Autodesk Inventor part; units mm, degrees
(part 2 of 2)
  arc A595 (0.658, -32.4933) -> (0.5633, -32.568) centre (0.66, -32.5933) ccw
  arc A596 (-0.2221, -33.5687) -> (-0.1304, -33.6297) centre (-0.13, -33.5297) ccw
  arc A597 (-0.5633, -32.568) -> (-0.2221, -33.5687) centre (6.5366, -30.706) ccw
  arc A598 (-0.5633, -32.568) -> (-0.658, -32.4933) centre (-0.66, -32.5933) ccw
  arc A599 (0.2221, -33.5687) -> (0.5633, -32.568) centre (-6.5366, -30.706) ccw
  arc A600 (0.1304, -33.6297) -> (0.2221, -33.5687) centre (0.13, -33.5297) ccw
  arc A601 (2.2033, -32.4252) -> (2.1123, -32.5043) centre (2.2101, -32.525) ccw
  arc A602 (1.3754, -33.5413) -> (1.4699, -33.5979) centre (1.4656, -33.498) ccw
  arc A603 (0.987, -32.5579) -> (1.3754, -33.5413) centre (7.9903, -30.3602) ccw
  arc A604 (0.987, -32.5579) -> (0.8889, -32.4878) centre (0.8916, -32.5878) ccw
  arc A605 (1.8191, -33.5202) -> (2.1123, -32.5043) centre (-5.0682, -30.9823) ccw
  arc A606 (1.7304, -33.5855) -> (1.8191, -33.5202) centre (1.7253, -33.4856) ccw
  arc A607 (3.7437, -32.2837) -> (3.6565, -32.3669) centre (3.7552, -32.383) ccw
  arc A608 (2.9698, -33.4379) -> (3.0669, -33.4899) centre (3.0578, -33.3903) ccw
  arc A609 (2.5351, -32.474) -> (2.9698, -33.4379) centre (9.4258, -29.9456) ccw
  arc A610 (2.5351, -32.474) -> (2.4337, -32.4088) centre (2.4412, -32.5085) ccw
  arc A611 (3.412, -33.3956) -> (3.6565, -32.3669) centre (-3.5883, -31.1883) ccw
  arc A612 (3.3265, -33.4651) -> (3.412, -33.3956) centre (3.3166, -33.3656) ccw
  arc A613 (5.2756, -32.069) -> (5.1924, -32.1563) centre (5.2918, -32.1676) ccw
  arc A614 (4.5575, -33.2587) -> (4.657, -33.306) centre (4.6431, -33.207) ccw
  arc A615 (4.0774, -32.3166) -> (4.5575, -33.2587) centre (10.84, -29.4632) ccw
  arc A616 (4.0774, -32.3166) -> (3.973, -32.2562) centre (3.9852, -32.3555) ccw
  arc A617 (4.9972, -33.1955) -> (5.1924, -32.1563) centre (-2.1002, -31.3237) ccw
  arc A618 (4.9151, -33.2689) -> (4.9972, -33.1955) centre (4.9005, -33.17) ccw
  arc A619 (6.7955, -31.7816) -> (6.7166, -31.8728) centre (6.8164, -31.8794) ccw
  arc A620 (6.1349, -33.0041) -> (6.2364, -33.0467) centre (6.2179, -32.9484) ccw
  arc A621 (5.6104, -32.086) -> (6.1349, -33.0041) centre (12.2297, -28.9141) ccw
  arc A622 (5.6104, -32.086) -> (5.5033, -32.0307) centre (5.5203, -32.1292) ccw
  arc A623 (6.571, -32.9201) -> (6.7166, -31.8728) centre (-0.6074, -31.3882) ccw
  arc A624 (6.4925, -32.9973) -> (6.571, -32.9201) centre (6.4732, -32.8992) ccw
  arc A625 (8.3, -31.4223) -> (8.2256, -31.5171) centre (8.3256, -31.519) ccw
  arc A626 (7.6983, -32.6749) -> (7.8018, -32.7125) centre (7.7786, -32.6152) ccw
  arc A627 (7.1308, -31.7827) -> (7.6983, -32.6749) centre (13.5916, -28.2994) ccw
  arc A628 (7.1308, -31.7827) -> (7.0212, -31.7325) centre (7.0428, -31.8302) ccw
  arc A629 (8.13, -32.5701) -> (8.2256, -31.5171) centre (0.8868, -31.3815) ccw
  arc A630 (8.0552, -32.651) -> (8.13, -32.5701) centre (8.0313, -32.5539) ccw
  arc A631 (9.7858, -30.9918) -> (9.7159, -31.09) centre (9.8159, -31.0871) ccw
  arc A632 (9.2443, -32.2715) -> (9.3495, -32.3042) centre (9.3217, -32.2082) ccw
  arc A633 (8.635, -31.4074) -> (9.2443, -32.2715) centre (14.9228, -27.6206) ccw
  arc A634 (8.635, -31.4074) -> (8.5231, -31.3625) centre (8.5493, -31.459) ccw
  arc A635 (9.6705, -32.1464) -> (9.7159, -31.09) centre (2.379, -31.3038) ccw
  arc A636 (9.5997, -32.2308) -> (9.6705, -32.1464) centre (9.5712, -32.1349) ccw
  arc A637 (11.2493, -30.491) -> (11.1842, -30.5925) centre (11.2839, -30.5848) ccw
  arc A638 (10.7694, -31.7951) -> (10.876, -31.8228) centre (10.8437, -31.7282) ccw
  arc A639 (10.1196, -30.961) -> (10.7694, -31.7951) centre (16.2201, -26.8793) ccw
  arc A640 (10.1196, -30.961) -> (10.0057, -30.9214) centre (10.0365, -31.0166) ccw
  arc A641 (11.1891, -31.6499) -> (11.1842, -30.5925) centre (3.8658, -31.1551) ccw
  arc A642 (11.1224, -31.7375) -> (11.1891, -31.6499) centre (11.0894, -31.6431) ccw
  arc A643 (12.6874, -29.9212) -> (12.6272, -30.0257) centre (12.7264, -30.0133) ccw
  arc A644 (12.2701, -31.2467) -> (12.3779, -31.2692) centre (12.3411, -31.1763) ccw
  arc A645 (11.5814, -30.4444) -> (12.2701, -31.2467) centre (17.4807, -26.0771) ccw
  arc A646 (11.5814, -30.4444) -> (11.4657, -30.4103) centre (11.501, -30.5039) ccw
  arc A647 (12.6824, -31.0816) -> (12.6272, -30.0257) centre (5.3439, -30.9359) ccw
  arc A648 (12.62, -31.1723) -> (12.6824, -31.0816) centre (12.5824, -31.0796) ccw
  arc A649 (14.0967, -29.2836) -> (14.0416, -29.3909) centre (14.1401, -29.3738) ccw
  arc A650 (13.743, -30.6275) -> (13.8517, -30.6449) centre (13.8105, -30.5537) ccw
  arc A651 (13.0168, -29.8588) -> (13.743, -30.6275) centre (18.7017, -25.2158) ccw
  arc A652 (13.0168, -29.8588) -> (12.8997, -29.8303) centre (12.9394, -29.9221) ccw
  arc A653 (14.147, -30.443) -> (14.0416, -29.3909) centre (6.8098, -30.6466) ccw
  arc A654 (14.0889, -30.5365) -> (14.147, -30.443) centre (14.047, -30.4457) ccw
  arc A655 (15.4741, -28.5797) -> (15.4242, -28.6894) centre (15.5218, -28.6677) ccw
  arc A656 (15.1847, -29.9389) -> (15.2941, -29.9511) centre (15.2487, -29.862) ccw
  arc A657 (14.4228, -29.2057) -> (15.1847, -29.9389) centre (19.8803, -24.2973) ccw
  arc A658 (14.4228, -29.2057) -> (14.3045, -29.1827) centre (14.3485, -29.2725) ccw
  arc A659 (15.5795, -29.7353) -> (15.4242, -28.6894) centre (8.2603, -30.2879) ccw
  arc A660 (15.5259, -29.8316) -> (15.5795, -29.7353) centre (15.4798, -29.7429) ccw
  arc A661 (16.8165, -27.8111) -> (16.7718, -27.923) centre (16.8682, -27.8966) ccw
  arc A662 (16.592, -29.1824) -> (16.702, -29.1894) centre (16.6523, -29.1026) ccw
  arc A663 (15.7962, -28.4863) -> (16.592, -29.1824) centre (21.0139, -23.3239) ccw
  arc A664 (15.7962, -28.4863) -> (15.6768, -28.469) centre (15.7251, -28.5566) ccw
  arc A665 (16.9767, -28.9603) -> (16.7718, -27.923) centre (9.6921, -29.8605) ccw
  arc A666 (16.9278, -29.059) -> (16.9767, -28.9603) centre (16.8775, -28.9726) ccw
  arc A667 (18.1207, -26.9794) -> (18.0814, -27.0934) centre (18.1765, -27.0624) ccw
  arc A668 (17.9618, -28.3599) -> (18.0719, -28.3616) centre (18.0182, -28.2773) ccw
  arc A669 (17.1337, -27.7024) -> (17.9618, -28.3599) centre (22.0999, -22.2976) ccw
  arc A670 (17.1337, -27.7024) -> (17.0137, -27.6909) centre (17.0661, -27.7761) ccw
  arc A671 (18.3355, -28.1198) -> (18.0814, -27.0934) centre (11.102, -29.3655) ccw
  arc A672 (18.2913, -28.2207) -> (18.3355, -28.1198) centre (18.2369, -28.1367) ccw
  arc A673 (19.384, -26.0866) -> (19.3501, -26.2023) centre (19.4436, -26.1669) ccw
  arc A674 (19.2909, -27.4731) -> (19.401, -27.4696) centre (19.3433, -27.3879) ccw
  arc A675 (18.4324, -26.8558) -> (19.2909, -27.4731) centre (23.1358, -21.2208) ccw
  arc A676 (18.4324, -26.8558) -> (18.312, -26.85) centre (18.3684, -26.9326) ccw
  arc A677 (19.6527, -27.2155) -> (19.3501, -26.2023) centre (12.4866, -28.804) ccw
  arc A678 (19.6134, -27.3184) -> (19.6527, -27.2155) centre (19.5551, -27.2371) ccw
  arc A679 (20.6033, -25.1348) -> (20.5749, -25.2519) centre (20.6666, -25.2121) ccw
  arc A680 (20.5763, -26.5241) -> (20.686, -26.5154) centre (20.6245, -26.4365) ccw
  arc A681 (19.6894, -25.9483) -> (20.5763, -26.5241) centre (24.1194, -20.0959) ccw
  arc A682 (19.6894, -25.9483) -> (19.5688, -25.9482) centre (19.6291, -26.0281) ccw
  arc A683 (20.9254, -26.2495) -> (20.5749, -25.2519) centre (13.8431, -28.1772) ccw
  arc A684 (20.891, -26.3542) -> (20.9254, -26.2495) centre (20.8289, -26.2758) ccw
  arc A685 (21.7759, -24.1259) -> (21.7532, -24.2444) centre (21.8429, -24.2002) ccw
  arc A686 (21.815, -25.515) -> (21.9243, -25.5011) centre (21.8591, -25.4252) ccw
  arc A687 (20.9018, -24.9821) -> (21.815, -25.515) centre (25.0482, -18.9255) ccw
  arc A688 (20.9018, -24.9821) -> (20.7813, -24.9877) centre (20.8453, -25.0646) ccw
  arc A689 (22.1507, -25.2241) -> (21.7532, -24.2444) centre (15.1681, -27.4867) ccw
  arc A690 (22.1213, -25.3303) -> (22.1507, -25.2241) centre (22.0556, -25.255) ccw
  arc A691 (22.8992, -23.0625) -> (22.8821, -23.1818) centre (22.9696, -23.1334) ccw
  arc A692 (23.0044, -24.4481) -> (23.1128, -24.429) centre (23.0441, -24.3563) ccw
  arc A693 (22.0668, -23.9592) -> (23.0044, -24.4481) centre (25.9204, -17.7122) ccw
  arc A694 (22.0668, -23.9592) -> (21.9468, -23.9706) centre (22.0143, -24.0443) ccw
  arc A695 (23.3258, -24.1416) -> (22.8821, -23.1818) centre (16.4588, -26.7338) ccw
  arc A696 (23.3015, -24.249) -> (23.3258, -24.1416) centre (23.2323, -24.1769) ccw
  arc A697 (23.9706, -21.9468) -> (23.9592, -22.0668) centre (24.0443, -22.0143) ccw
  arc A698 (24.1416, -23.3258) -> (24.249, -23.3015) centre (24.1769, -23.2323) ccw
  arc A699 (23.1818, -22.8821) -> (24.1416, -23.3258) centre (26.7338, -16.4588) ccw
  arc A700 (23.1818, -22.8821) -> (23.0625, -22.8992) centre (23.1334, -22.9696) ccw
  arc A701 (24.4481, -23.0044) -> (23.9592, -22.0668) centre (17.7122, -25.9204) ccw
  arc A702 (24.429, -23.1128) -> (24.4481, -23.0044) centre (24.3563, -23.0441) ccw
  arc A703 (24.9877, -20.7813) -> (24.9821, -20.9018) centre (25.0646, -20.8453) ccw
  arc A704 (25.2241, -22.1507) -> (25.3303, -22.1213) centre (25.255, -22.0556) ccw
  arc A705 (24.2444, -21.7532) -> (25.2241, -22.1507) centre (27.4867, -15.1681) ccw
  arc A706 (24.2444, -21.7532) -> (24.1259, -21.7759) centre (24.2002, -21.8429) ccw
  arc A707 (25.515, -21.815) -> (24.9821, -20.9018) centre (18.9255, -25.0482) ccw
  arc A708 (25.5011, -21.9243) -> (25.515, -21.815) centre (25.4252, -21.8591) ccw
  arc A709 (25.9482, -19.5688) -> (25.9483, -19.6894) centre (26.0281, -19.6291) ccw
  arc A710 (26.2495, -20.9254) -> (26.3542, -20.891) centre (26.2758, -20.8289) ccw
  arc A711 (25.2519, -20.5749) -> (26.2495, -20.9254) centre (28.1772, -13.8431) ccw
  arc A712 (25.2519, -20.5749) -> (25.1348, -20.6033) centre (25.2121, -20.6666) ccw
  arc A713 (26.5241, -20.5763) -> (25.9483, -19.6894) centre (20.0959, -24.1194) ccw
  arc A714 (26.5154, -20.686) -> (26.5241, -20.5763) centre (26.4365, -20.6245) ccw
  arc A715 (26.85, -18.312) -> (26.8558, -18.4324) centre (26.9326, -18.3684) ccw
  arc A716 (27.2155, -19.6527) -> (27.3184, -19.6134) centre (27.2371, -19.5551) ccw
  arc A717 (26.2023, -19.3501) -> (27.2155, -19.6527) centre (28.804, -12.4866) ccw
  arc A718 (26.2023, -19.3501) -> (26.0866, -19.384) centre (26.1669, -19.4436) ccw
  arc A719 (27.4731, -19.2909) -> (26.8558, -18.4324) centre (21.2208, -23.1358) ccw
  arc A720 (27.4696, -19.401) -> (27.4731, -19.2909) centre (27.3879, -19.3433) ccw
  arc A721 (27.6909, -17.0137) -> (27.7024, -17.1337) centre (27.7761, -17.0661) ccw
  arc A722 (28.1198, -18.3355) -> (28.2207, -18.2913) centre (28.1367, -18.2369) ccw
  arc A723 (27.0934, -18.0814) -> (28.1198, -18.3355) centre (29.3655, -11.102) ccw
  arc A724 (27.0934, -18.0814) -> (26.9794, -18.1207) centre (27.0624, -18.1765) ccw
  arc A725 (28.3599, -17.9618) -> (27.7024, -17.1337) centre (22.2976, -22.0999) ccw
  arc A726 (28.3616, -18.0719) -> (28.3599, -17.9618) centre (28.2773, -18.0182) ccw
  arc A727 (28.469, -15.6768) -> (28.4863, -15.7962) centre (28.5566, -15.7251) ccw
  arc A728 (28.9603, -16.9767) -> (29.059, -16.9278) centre (28.9726, -16.8775) ccw
  arc A729 (27.923, -16.7718) -> (28.9603, -16.9767) centre (29.8605, -9.6921) ccw
  arc A730 (27.923, -16.7718) -> (27.8111, -16.8165) centre (27.8966, -16.8682) ccw
  arc A731 (29.1824, -16.592) -> (28.4863, -15.7962) centre (23.3239, -21.0139) ccw
  arc A732 (29.1894, -16.702) -> (29.1824, -16.592) centre (29.1026, -16.6523) ccw
  arc A733 (29.1827, -14.3045) -> (29.2057, -14.4228) centre (29.2725, -14.3485) ccw
  arc A734 (29.7353, -15.5795) -> (29.8316, -15.5259) centre (29.7429, -15.4798) ccw
  arc A735 (28.6894, -15.4242) -> (29.7353, -15.5795) centre (30.2879, -8.2603) ccw
  arc A736 (28.6894, -15.4242) -> (28.5797, -15.4741) centre (28.6677, -15.5218) ccw
  arc A737 (29.9389, -15.1847) -> (29.2057, -14.4228) centre (24.2973, -19.8803) ccw
  arc A738 (29.9511, -15.2941) -> (29.9389, -15.1847) centre (29.862, -15.2487) ccw
  arc A739 (29.8303, -12.8997) -> (29.8588, -13.0168) centre (29.9221, -12.9394) ccw
  arc A740 (30.443, -14.147) -> (30.5365, -14.0889) centre (30.4457, -14.047) ccw
  arc A741 (29.3909, -14.0416) -> (30.443, -14.147) centre (30.6466, -6.8098) ccw
  arc A742 (29.3909, -14.0416) -> (29.2836, -14.0967) centre (29.3738, -14.1401) ccw
  arc A743 (30.6275, -13.743) -> (29.8588, -13.0168) centre (25.2158, -18.7017) ccw
  arc A744 (30.6449, -13.8517) -> (30.6275, -13.743) centre (30.5537, -13.8105) ccw
  arc A745 (30.4103, -11.4657) -> (30.4444, -11.5814) centre (30.5039, -11.501) ccw
  arc A746 (31.0816, -12.6824) -> (31.1723, -12.62) centre (31.0796, -12.5824) ccw
  arc A747 (30.0257, -12.6272) -> (31.0816, -12.6824) centre (30.9359, -5.3439) ccw
  arc A748 (30.0257, -12.6272) -> (29.9212, -12.6874) centre (30.0133, -12.7264) ccw
  arc A749 (31.2467, -12.2701) -> (30.4444, -11.5814) centre (26.0771, -17.4807) ccw
  arc A750 (31.2692, -12.3779) -> (31.2467, -12.2701) centre (31.1763, -12.3411) ccw
  arc A751 (30.9214, -10.0057) -> (30.961, -10.1196) centre (31.0166, -10.0365) ccw
  arc A752 (31.6499, -11.1891) -> (31.7375, -11.1224) centre (31.6431, -11.0894) ccw
  arc A753 (30.5925, -11.1842) -> (31.6499, -11.1891) centre (31.1551, -3.8658) ccw
  arc A754 (30.5925, -11.1842) -> (30.491, -11.2493) centre (30.5848, -11.2839) ccw
  arc A755 (31.7951, -10.7694) -> (30.961, -10.1196) centre (26.8793, -16.2201) ccw
  arc A756 (31.8228, -10.876) -> (31.7951, -10.7694) centre (31.7282, -10.8437) ccw
  arc A757 (31.3625, -8.5231) -> (31.4074, -8.635) centre (31.459, -8.5493) ccw
  arc A758 (32.1464, -9.6705) -> (32.2308, -9.5997) centre (32.1349, -9.5712) ccw
  arc A759 (31.09, -9.7159) -> (32.1464, -9.6705) centre (31.3038, -2.379) ccw
  arc A760 (31.09, -9.7159) -> (30.9918, -9.7858) centre (31.0871, -9.8159) ccw
  arc A761 (32.2715, -9.2443) -> (31.4074, -8.635) centre (27.6206, -14.9228) ccw
  arc A762 (32.3042, -9.3495) -> (32.2715, -9.2443) centre (32.2082, -9.3217) ccw
  arc A763 (31.7325, -7.0212) -> (31.7827, -7.1308) centre (31.8302, -7.0428) ccw
  arc A764 (32.5701, -8.13) -> (32.651, -8.0552) centre (32.5539, -8.0313) ccw
  arc A765 (31.5171, -8.2256) -> (32.5701, -8.13) centre (31.3815, -0.8868) ccw
  arc A766 (31.5171, -8.2256) -> (31.4223, -8.3) centre (31.519, -8.3256) ccw
  arc A767 (32.6749, -7.6983) -> (31.7827, -7.1308) centre (28.2994, -13.5916) ccw
  arc A768 (32.7125, -7.8018) -> (32.6749, -7.6983) centre (32.6152, -7.7786) ccw
  arc A769 (32.0307, -5.5033) -> (32.086, -5.6104) centre (32.1292, -5.5203) ccw
  arc A770 (32.9201, -6.571) -> (32.9973, -6.4925) centre (32.8992, -6.4732) ccw
  arc A771 (31.8728, -6.7166) -> (32.9201, -6.571) centre (31.3882, 0.6074) ccw
  arc A772 (31.8728, -6.7166) -> (31.7816, -6.7955) centre (31.8794, -6.8164) ccw
  arc A773 (33.0041, -6.1349) -> (32.086, -5.6104) centre (28.9141, -12.2297) ccw
  arc A774 (33.0467, -6.2364) -> (33.0041, -6.1349) centre (32.9484, -6.2179) ccw
  arc A775 (32.2562, -3.973) -> (32.3166, -4.0774) centre (32.3555, -3.9852) ccw
  arc A776 (33.1955, -4.9972) -> (33.2689, -4.9151) centre (33.17, -4.9005) ccw
  arc A777 (32.1563, -5.1924) -> (33.1955, -4.9972) centre (31.3237, 2.1002) ccw
  arc A778 (32.1563, -5.1924) -> (32.069, -5.2756) centre (32.1676, -5.2918) ccw
  arc A779 (33.2587, -4.5575) -> (32.3166, -4.0774) centre (29.4632, -10.84) ccw
  arc A780 (33.306, -4.657) -> (33.2587, -4.5575) centre (33.207, -4.6431) ccw
  arc A781 (32.4088, -2.4337) -> (32.474, -2.5351) centre (32.5085, -2.4412) ccw
  arc A782 (33.3956, -3.412) -> (33.4651, -3.3265) centre (33.3656, -3.3166) ccw
  arc A783 (32.3669, -3.6565) -> (33.3956, -3.412) centre (31.1883, 3.5883) ccw
  arc A784 (32.3669, -3.6565) -> (32.2837, -3.7437) centre (32.383, -3.7552) ccw
  arc A785 (33.4379, -2.9698) -> (32.474, -2.5351) centre (29.9456, -9.4258) ccw
  arc A786 (33.4899, -3.0669) -> (33.4379, -2.9698) centre (33.3903, -3.0578) ccw
  arc A787 (32.4878, -0.8889) -> (32.5579, -0.987) centre (32.5878, -0.8916) ccw
  arc A788 (33.5202, -1.8191) -> (33.5855, -1.7304) centre (33.4856, -1.7253) ccw
  arc A789 (32.5043, -2.1123) -> (33.5202, -1.8191) centre (30.9823, 5.0682) ccw
  arc A790 (32.5043, -2.1123) -> (32.4252, -2.2033) centre (32.525, -2.2101) ccw
  arc A791 (33.5413, -1.3754) -> (32.5579, -0.987) centre (30.3602, -7.9903) ccw
  arc A792 (33.5979, -1.4699) -> (33.5413, -1.3754) centre (33.498, -1.4656) ccw
  arc A793 (30.6449, 13.8517) -> (30.5365, 14.0889) centre (0, 0) ccw
  arc A794 (31.2692, 12.3779) -> (31.1723, 12.62) centre (0, 0) ccw
  arc A795 (31.8228, 10.876) -> (31.7375, 11.1224) centre (0, 0) ccw
  arc A796 (32.3042, 9.3495) -> (32.2308, 9.5997) centre (0, 0) ccw
  arc A797 (29.9212, 12.6874) -> (29.8303, 12.8997) centre (0, 0) ccw
  arc A798 (30.491, 11.2493) -> (30.4103, 11.4657) centre (0, 0) ccw
  arc A799 (30.9918, 9.7858) -> (30.9214, 10.0057) centre (0, 0) ccw
  arc A800 (31.4223, 8.3) -> (31.3625, 8.5231) centre (0, 0) ccw
  arc A801 (32.7125, 7.8018) -> (32.651, 8.0552) centre (0, 0) ccw
  arc A802 (33.0467, 6.2364) -> (32.9973, 6.4925) centre (0, 0) ccw
  arc A803 (33.306, 4.657) -> (33.2689, 4.9151) centre (0, 0) ccw
  arc A804 (33.4899, 3.0669) -> (33.4651, 3.3265) centre (0, 0) ccw
  arc A805 (33.5979, 1.4699) -> (33.5855, 1.7304) centre (0, 0) ccw
  arc A806 (33.6297, -0.1304) -> (33.6297, 0.1304) centre (0, 0) ccw
  arc A807 (33.5855, -1.7304) -> (33.5979, -1.4699) centre (0, 0) ccw
  arc A808 (33.4651, -3.3265) -> (33.4899, -3.0669) centre (0, 0) ccw
  arc A809 (31.7816, 6.7955) -> (31.7325, 7.0212) centre (0, 0) ccw
  arc A810 (32.069, 5.2756) -> (32.0307, 5.5033) centre (0, 0) ccw
  arc A811 (32.2837, 3.7437) -> (32.2562, 3.973) centre (0, 0) ccw
  arc A812 (32.4252, 2.2033) -> (32.4088, 2.4337) centre (0, 0) ccw
  arc A813 (32.4933, 0.658) -> (32.4878, 0.8889) centre (0, 0) ccw
  arc A814 (32.4878, -0.8889) -> (32.4933, -0.658) centre (0, 0) ccw
  arc A815 (32.4088, -2.4337) -> (32.4252, -2.2033) centre (0, 0) ccw
  arc A816 (32.2562, -3.973) -> (32.2837, -3.7437) centre (0, 0) ccw
  arc A817 (32.0307, -5.5033) -> (32.069, -5.2756) centre (0, 0) ccw
  arc A818 (31.7325, -7.0212) -> (31.7816, -6.7955) centre (0, 0) ccw
  arc A819 (31.3625, -8.5231) -> (31.4223, -8.3) centre (0, 0) ccw
  arc A820 (30.9214, -10.0057) -> (30.9918, -9.7858) centre (0, 0) ccw
  arc A821 (30.4103, -11.4657) -> (30.491, -11.2493) centre (0, 0) ccw
  arc A822 (29.8303, -12.8997) -> (29.9212, -12.6874) centre (0, 0) ccw
  arc A823 (29.1827, -14.3045) -> (29.2836, -14.0967) centre (0, 0) ccw
  arc A824 (28.469, -15.6768) -> (28.5797, -15.4741) centre (0, 0) ccw
  arc A825 (27.6909, -17.0137) -> (27.8111, -16.8165) centre (0, 0) ccw
  arc A826 (26.85, -18.312) -> (26.9794, -18.1207) centre (0, 0) ccw
  arc A827 (25.9482, -19.5688) -> (26.0866, -19.384) centre (0, 0) ccw
  arc A828 (24.9877, -20.7813) -> (25.1348, -20.6033) centre (0, 0) ccw
  arc A829 (23.9706, -21.9468) -> (24.1259, -21.7759) centre (0, 0) ccw
  arc A830 (22.8992, -23.0625) -> (23.0625, -22.8992) centre (0, 0) ccw
  arc A831 (33.2689, -4.9151) -> (33.306, -4.657) centre (0, 0) ccw
  arc A832 (32.9973, -6.4925) -> (33.0467, -6.2364) centre (0, 0) ccw
  arc A833 (32.651, -8.0552) -> (32.7125, -7.8018) centre (0, 0) ccw
  arc A834 (32.2308, -9.5997) -> (32.3042, -9.3495) centre (0, 0) ccw
  arc A835 (31.7375, -11.1224) -> (31.8228, -10.876) centre (0, 0) ccw
  arc A836 (31.1723, -12.62) -> (31.2692, -12.3779) centre (0, 0) ccw
  arc A837 (30.5365, -14.0889) -> (30.6449, -13.8517) centre (0, 0) ccw
  arc A838 (29.8316, -15.5259) -> (29.9511, -15.2941) centre (0, 0) ccw
  arc A839 (29.059, -16.9278) -> (29.1894, -16.702) centre (0, 0) ccw
  arc A840 (28.2207, -18.2913) -> (28.3616, -18.0719) centre (0, 0) ccw
  arc A841 (27.3184, -19.6134) -> (27.4696, -19.401) centre (0, 0) ccw
  arc A842 (26.3542, -20.891) -> (26.5154, -20.686) centre (0, 0) ccw
  arc A843 (25.3303, -22.1213) -> (25.5011, -21.9243) centre (0, 0) ccw
  arc A844 (24.249, -23.3015) -> (24.429, -23.1128) centre (0, 0) ccw
  arc A845 (23.1128, -24.429) -> (23.3015, -24.249) centre (0, 0) ccw
  arc A846 (21.9243, -25.5011) -> (22.1213, -25.3303) centre (0, 0) ccw
  arc A847 (20.686, -26.5154) -> (20.891, -26.3542) centre (0, 0) ccw
  arc A848 (19.401, -27.4696) -> (19.6134, -27.3184) centre (0, 0) ccw
  arc A849 (18.0719, -28.3616) -> (18.2913, -28.2207) centre (0, 0) ccw
  arc A850 (16.702, -29.1894) -> (16.9278, -29.059) centre (0, 0) ccw
  arc A851 (15.2941, -29.9511) -> (15.5259, -29.8316) centre (0, 0) ccw
  arc A852 (13.8517, -30.6449) -> (14.0889, -30.5365) centre (0, 0) ccw
  arc A853 (12.3779, -31.2692) -> (12.62, -31.1723) centre (0, 0) ccw
  arc A854 (10.876, -31.8228) -> (11.1224, -31.7375) centre (0, 0) ccw
  arc A855 (9.3495, -32.3042) -> (9.5997, -32.2308) centre (0, 0) ccw
  arc A856 (7.8018, -32.7125) -> (8.0552, -32.651) centre (0, 0) ccw
  arc A857 (6.2364, -33.0467) -> (6.4925, -32.9973) centre (0, 0) ccw
  arc A858 (4.657, -33.306) -> (4.9151, -33.2689) centre (0, 0) ccw
  arc A859 (3.0669, -33.4899) -> (3.3265, -33.4651) centre (0, 0) ccw
  arc A860 (1.4699, -33.5979) -> (1.7304, -33.5855) centre (0, 0) ccw
  arc A861 (21.7759, -24.1259) -> (21.9468, -23.9706) centre (0, 0) ccw
  arc A862 (20.6033, -25.1348) -> (20.7813, -24.9877) centre (0, 0) ccw
  arc A863 (19.384, -26.0866) -> (19.5688, -25.9482) centre (0, 0) ccw
  arc A864 (18.1207, -26.9794) -> (18.312, -26.85) centre (0, 0) ccw
  arc A865 (16.8165, -27.8111) -> (17.0137, -27.6909) centre (0, 0) ccw
  arc A866 (15.4741, -28.5797) -> (15.6768, -28.469) centre (0, 0) ccw
  arc A867 (14.0967, -29.2836) -> (14.3045, -29.1827) centre (0, 0) ccw
  arc A868 (12.6874, -29.9212) -> (12.8997, -29.8303) centre (0, 0) ccw
  arc A869 (11.2493, -30.491) -> (11.4657, -30.4103) centre (0, 0) ccw
  arc A870 (9.7858, -30.9918) -> (10.0057, -30.9214) centre (0, 0) ccw
  arc A871 (8.3, -31.4223) -> (8.5231, -31.3625) centre (0, 0) ccw
  arc A872 (6.7955, -31.7816) -> (7.0212, -31.7325) centre (0, 0) ccw
  arc A873 (5.2756, -32.069) -> (5.5033, -32.0307) centre (0, 0) ccw
  arc A874 (3.7437, -32.2837) -> (3.973, -32.2562) centre (0, 0) ccw
  arc A875 (2.2033, -32.4252) -> (2.4337, -32.4088) centre (0, 0) ccw
  arc A876 (0.658, -32.4933) -> (0.8889, -32.4878) centre (0, 0) ccw
  arc A877 (-0.8889, -32.4878) -> (-0.658, -32.4933) centre (0, 0) ccw
  arc A878 (-0.1304, -33.6297) -> (0.1304, -33.6297) centre (0, 0) ccw
  arc A879 (-1.7304, -33.5855) -> (-1.4699, -33.5979) centre (0, 0) ccw
  arc A880 (-3.3265, -33.4651) -> (-3.0669, -33.4899) centre (0, 0) ccw
  arc A881 (-4.9151, -33.2689) -> (-4.657, -33.306) centre (0, 0) ccw
  arc A882 (-6.4925, -32.9973) -> (-6.2364, -33.0467) centre (0, 0) ccw
  arc A883 (-8.0552, -32.651) -> (-7.8018, -32.7125) centre (0, 0) ccw
  arc A884 (-9.5997, -32.2308) -> (-9.3495, -32.3042) centre (0, 0) ccw
  arc A885 (-11.1224, -31.7375) -> (-10.876, -31.8228) centre (0, 0) ccw
  arc A886 (-12.62, -31.1723) -> (-12.3779, -31.2692) centre (0, 0) ccw
  arc A887 (-14.0889, -30.5365) -> (-13.8517, -30.6449) centre (0, 0) ccw
  arc A888 (-15.5259, -29.8316) -> (-15.2941, -29.9511) centre (0, 0) ccw
  arc A889 (-16.9278, -29.059) -> (-16.702, -29.1894) centre (0, 0) ccw
  arc A890 (-18.2913, -28.2207) -> (-18.0719, -28.3616) centre (0, 0) ccw
  arc A891 (-19.6134, -27.3184) -> (-19.401, -27.4696) centre (0, 0) ccw
  arc A892 (-20.891, -26.3542) -> (-20.686, -26.5154) centre (0, 0) ccw
  arc A893 (-22.1213, -25.3303) -> (-21.9243, -25.5011) centre (0, 0) ccw
  arc A894 (-23.3015, -24.249) -> (-23.1128, -24.429) centre (0, 0) ccw
  arc A895 (-24.429, -23.1128) -> (-24.249, -23.3015) centre (0, 0) ccw
  arc A896 (-25.5011, -21.9243) -> (-25.3303, -22.1213) centre (0, 0) ccw
  arc A897 (-26.5154, -20.686) -> (-26.3542, -20.891) centre (0, 0) ccw
  arc A898 (-27.4696, -19.401) -> (-27.3184, -19.6134) centre (0, 0) ccw
  arc A899 (-28.3616, -18.0719) -> (-28.2207, -18.2913) centre (0, 0) ccw
  arc A900 (-29.1894, -16.702) -> (-29.059, -16.9278) centre (0, 0) ccw
  arc A901 (-2.4337, -32.4088) -> (-2.2033, -32.4252) centre (0, 0) ccw
  arc A902 (-3.973, -32.2562) -> (-3.7437, -32.2837) centre (0, 0) ccw
  arc A903 (-5.5033, -32.0307) -> (-5.2756, -32.069) centre (0, 0) ccw
  arc A904 (-7.0212, -31.7325) -> (-6.7955, -31.7816) centre (0, 0) ccw
  arc A905 (-8.5231, -31.3625) -> (-8.3, -31.4223) centre (0, 0) ccw
  arc A906 (-10.0057, -30.9214) -> (-9.7858, -30.9918) centre (0, 0) ccw
  arc A907 (-11.4657, -30.4103) -> (-11.2493, -30.491) centre (0, 0) ccw
  arc A908 (-12.8997, -29.8303) -> (-12.6874, -29.9212) centre (0, 0) ccw
  arc A909 (-14.3045, -29.1827) -> (-14.0967, -29.2836) centre (0, 0) ccw
  arc A910 (-15.6768, -28.469) -> (-15.4741, -28.5797) centre (0, 0) ccw
  arc A911 (-17.0137, -27.6909) -> (-16.8165, -27.8111) centre (0, 0) ccw
  arc A912 (-18.312, -26.85) -> (-18.1207, -26.9794) centre (0, 0) ccw
  arc A913 (-19.5688, -25.9482) -> (-19.384, -26.0866) centre (0, 0) ccw
  arc A914 (-20.7813, -24.9877) -> (-20.6033, -25.1348) centre (0, 0) ccw
  arc A915 (-21.9468, -23.9706) -> (-21.7759, -24.1259) centre (0, 0) ccw
  arc A916 (-23.0625, -22.8992) -> (-22.8992, -23.0625) centre (0, 0) ccw
  arc A917 (-24.1259, -21.7759) -> (-23.9706, -21.9468) centre (0, 0) ccw
  arc A918 (-25.1348, -20.6033) -> (-24.9877, -20.7813) centre (0, 0) ccw
  arc A919 (-26.0866, -19.384) -> (-25.9482, -19.5688) centre (0, 0) ccw
  arc A920 (-26.9794, -18.1207) -> (-26.85, -18.312) centre (0, 0) ccw
  arc A921 (-27.8111, -16.8165) -> (-27.6909, -17.0137) centre (0, 0) ccw
  arc A922 (-28.5797, -15.4741) -> (-28.469, -15.6768) centre (0, 0) ccw
  arc A923 (-29.2836, -14.0967) -> (-29.1827, -14.3045) centre (0, 0) ccw
  arc A924 (-29.9212, -12.6874) -> (-29.8303, -12.8997) centre (0, 0) ccw
  arc A925 (-30.491, -11.2493) -> (-30.4103, -11.4657) centre (0, 0) ccw
  arc A926 (-29.9511, -15.2941) -> (-29.8316, -15.5259) centre (0, 0) ccw
  arc A927 (-30.6449, -13.8517) -> (-30.5365, -14.0889) centre (0, 0) ccw
  arc A928 (-31.2692, -12.3779) -> (-31.1723, -12.62) centre (0, 0) ccw
  arc A929 (-31.8228, -10.876) -> (-31.7375, -11.1224) centre (0, 0) ccw
  arc A930 (-32.3042, -9.3495) -> (-32.2308, -9.5997) centre (0, 0) ccw
  arc A931 (-32.7125, -7.8018) -> (-32.651, -8.0552) centre (0, 0) ccw
  arc A932 (-33.0467, -6.2364) -> (-32.9973, -6.4925) centre (0, 0) ccw
  arc A933 (-33.306, -4.657) -> (-33.2689, -4.9151) centre (0, 0) ccw
  arc A934 (-33.4899, -3.0669) -> (-33.4651, -3.3265) centre (0, 0) ccw
  arc A935 (-33.5979, -1.4699) -> (-33.5855, -1.7304) centre (0, 0) ccw
  arc A936 (-33.6297, 0.1304) -> (-33.6297, -0.1304) centre (0, 0) ccw
  arc A937 (-33.5855, 1.7304) -> (-33.5979, 1.4699) centre (0, 0) ccw
  arc A938 (-33.4651, 3.3265) -> (-33.4899, 3.0669) centre (0, 0) ccw
  arc A939 (-33.2689, 4.9151) -> (-33.306, 4.657) centre (0, 0) ccw
  arc A940 (-32.9973, 6.4925) -> (-33.0467, 6.2364) centre (0, 0) ccw
  arc A941 (-32.651, 8.0552) -> (-32.7125, 7.8018) centre (0, 0) ccw
  arc A942 (-32.2308, 9.5997) -> (-32.3042, 9.3495) centre (0, 0) ccw
  arc A943 (-31.7375, 11.1224) -> (-31.8228, 10.876) centre (0, 0) ccw
  arc A944 (-31.1723, 12.62) -> (-31.2692, 12.3779) centre (0, 0) ccw
  arc A945 (-30.5365, 14.0889) -> (-30.6449, 13.8517) centre (0, 0) ccw
  arc A946 (-29.8316, 15.5259) -> (-29.9511, 15.2941) centre (0, 0) ccw
  arc A947 (-29.059, 16.9278) -> (-29.1894, 16.702) centre (0, 0) ccw
  arc A948 (-28.2207, 18.2913) -> (-28.3616, 18.0719) centre (0, 0) ccw
  arc A949 (-27.3184, 19.6134) -> (-27.4696, 19.401) centre (0, 0) ccw
  arc A950 (-26.3542, 20.891) -> (-26.5154, 20.686) centre (0, 0) ccw
  arc A951 (-30.9918, -9.7858) -> (-30.9214, -10.0057) centre (0, 0) ccw
  arc A952 (-31.4223, -8.3) -> (-31.3625, -8.5231) centre (0, 0) ccw
  arc A953 (-31.7816, -6.7955) -> (-31.7325, -7.0212) centre (0, 0) ccw
  arc A954 (-32.069, -5.2756) -> (-32.0307, -5.5033) centre (0, 0) ccw
  arc A955 (-32.2837, -3.7437) -> (-32.2562, -3.973) centre (0, 0) ccw
  arc A956 (-32.4252, -2.2033) -> (-32.4088, -2.4337) centre (0, 0) ccw
  arc A957 (-32.4933, -0.658) -> (-32.4878, -0.8889) centre (0, 0) ccw
  arc A958 (-32.4878, 0.8889) -> (-32.4933, 0.658) centre (0, 0) ccw
  arc A959 (-32.4088, 2.4337) -> (-32.4252, 2.2033) centre (0, 0) ccw
  arc A960 (-32.2562, 3.973) -> (-32.2837, 3.7437) centre (0, 0) ccw
  arc A961 (-32.0307, 5.5033) -> (-32.069, 5.2756) centre (0, 0) ccw
  arc A962 (-31.7325, 7.0212) -> (-31.7816, 6.7955) centre (0, 0) ccw
  arc A963 (-31.3625, 8.5231) -> (-31.4223, 8.3) centre (0, 0) ccw
  arc A964 (-30.9214, 10.0057) -> (-30.9918, 9.7858) centre (0, 0) ccw
  arc A965 (-30.4103, 11.4657) -> (-30.491, 11.2493) centre (0, 0) ccw
  arc A966 (-29.8303, 12.8997) -> (-29.9212, 12.6874) centre (0, 0) ccw
  arc A967 (-29.1827, 14.3045) -> (-29.2836, 14.0967) centre (0, 0) ccw
  arc A968 (-28.469, 15.6768) -> (-28.5797, 15.4741) centre (0, 0) ccw
  arc A969 (-27.6909, 17.0137) -> (-27.8111, 16.8165) centre (0, 0) ccw
  arc A970 (-26.85, 18.312) -> (-26.9794, 18.1207) centre (0, 0) ccw
  arc A971 (-25.9482, 19.5688) -> (-26.0866, 19.384) centre (0, 0) ccw
  arc A972 (-24.9877, 20.7813) -> (-25.1348, 20.6033) centre (0, 0) ccw
  arc A973 (-23.9706, 21.9468) -> (-24.1259, 21.7759) centre (0, 0) ccw
  arc A974 (12.8997, 29.8303) -> (12.6874, 29.9212) centre (0, 0) ccw
  arc A975 (11.4657, 30.4103) -> (11.2493, 30.491) centre (0, 0) ccw
  arc A976 (10.0057, 30.9214) -> (9.7858, 30.9918) centre (0, 0) ccw
  arc A977 (8.5231, 31.3625) -> (8.3, 31.4223) centre (0, 0) ccw
  arc A978 (7.0212, 31.7325) -> (6.7955, 31.7816) centre (0, 0) ccw
  arc A979 (5.5033, 32.0307) -> (5.2756, 32.069) centre (0, 0) ccw
  arc A980 (3.973, 32.2562) -> (3.7437, 32.2837) centre (0, 0) ccw
  arc A981 (2.4337, 32.4088) -> (2.2033, 32.4252) centre (0, 0) ccw
  arc A982 (0.8889, 32.4878) -> (0.658, 32.4933) centre (0, 0) ccw
  arc A983 (-0.658, 32.4933) -> (-0.8889, 32.4878) centre (0, 0) ccw
  arc A984 (-2.2033, 32.4252) -> (-2.4337, 32.4088) centre (0, 0) ccw
  arc A985 (-3.7437, 32.2837) -> (-3.973, 32.2562) centre (0, 0) ccw
  arc A986 (-5.2756, 32.069) -> (-5.5033, 32.0307) centre (0, 0) ccw
  arc A987 (-6.7955, 31.7816) -> (-7.0212, 31.7325) centre (0, 0) ccw
  arc A988 (-8.3, 31.4223) -> (-8.5231, 31.3625) centre (0, 0) ccw
  arc A989 (-9.7858, 30.9918) -> (-10.0057, 30.9214) centre (0, 0) ccw
  arc A990 (-11.2493, 30.491) -> (-11.4657, 30.4103) centre (0, 0) ccw
  arc A991 (-12.6874, 29.9212) -> (-12.8997, 29.8303) centre (0, 0) ccw
  arc A992 (-14.0967, 29.2836) -> (-14.3045, 29.1827) centre (0, 0) ccw
  arc A993 (-15.4741, 28.5797) -> (-15.6768, 28.469) centre (0, 0) ccw
  arc A994 (-16.8165, 27.8111) -> (-17.0137, 27.6909) centre (0, 0) ccw
  arc A995 (-18.1207, 26.9794) -> (-18.312, 26.85) centre (0, 0) ccw
  arc A996 (-19.384, 26.0866) -> (-19.5688, 25.9482) centre (0, 0) ccw
  arc A997 (-20.6033, 25.1348) -> (-20.7813, 24.9877) centre (0, 0) ccw
  arc A998 (-21.7759, 24.1259) -> (-21.9468, 23.9706) centre (0, 0) ccw
  arc A999 (-22.8992, 23.0625) -> (-23.0625, 22.8992) centre (0, 0) ccw
  arc A1000 (12.62, 31.1723) -> (12.3779, 31.2692) centre (0, 0) ccw
  arc A1001 (11.1224, 31.7375) -> (10.876, 31.8228) centre (0, 0) ccw
  arc A1002 (9.5997, 32.2308) -> (9.3495, 32.3042) centre (0, 0) ccw
  arc A1003 (8.0552, 32.651) -> (7.8018, 32.7125) centre (0, 0) ccw
  arc A1004 (6.4925, 32.9973) -> (6.2364, 33.0467) centre (0, 0) ccw
  arc A1005 (4.9151, 33.2689) -> (4.657, 33.306) centre (0, 0) ccw
  arc A1006 (3.3265, 33.4651) -> (3.0669, 33.4899) centre (0, 0) ccw
  arc A1007 (1.7304, 33.5855) -> (1.4699, 33.5979) centre (0, 0) ccw
  arc A1008 (0.1304, 33.6297) -> (-0.1304, 33.6297) centre (0, 0) ccw
  arc A1009 (-1.4699, 33.5979) -> (-1.7304, 33.5855) centre (0, 0) ccw
  arc A1010 (-3.0669, 33.4899) -> (-3.3265, 33.4651) centre (0, 0) ccw
  arc A1011 (-4.657, 33.306) -> (-4.9151, 33.2689) centre (0, 0) ccw
  arc A1012 (-6.2364, 33.0467) -> (-6.4925, 32.9973) centre (0, 0) ccw
  arc A1013 (-7.8018, 32.7125) -> (-8.0552, 32.651) centre (0, 0) ccw
  arc A1014 (-9.3495, 32.3042) -> (-9.5997, 32.2308) centre (0, 0) ccw
  arc A1015 (-10.876, 31.8228) -> (-11.1224, 31.7375) centre (0, 0) ccw
  arc A1016 (-12.3779, 31.2692) -> (-12.62, 31.1723) centre (0, 0) ccw
  arc A1017 (-13.8517, 30.6449) -> (-14.0889, 30.5365) centre (0, 0) ccw
  arc A1018 (-15.2941, 29.9511) -> (-15.5259, 29.8316) centre (0, 0) ccw
  arc A1019 (-16.702, 29.1894) -> (-16.9278, 29.059) centre (0, 0) ccw
  arc A1020 (-18.0719, 28.3616) -> (-18.2913, 28.2207) centre (0, 0) ccw
  arc A1021 (-19.401, 27.4696) -> (-19.6134, 27.3184) centre (0, 0) ccw
  arc A1022 (-20.686, 26.5154) -> (-20.891, 26.3542) centre (0, 0) ccw
  arc A1023 (-21.9243, 25.5011) -> (-22.1213, 25.3303) centre (0, 0) ccw
  arc A1024 (-23.1128, 24.429) -> (-23.3015, 24.249) centre (0, 0) ccw
  arc A1025 (-24.249, 23.3015) -> (-24.429, 23.1128) centre (0, 0) ccw
  arc A1026 (-25.3303, 22.1213) -> (-25.5011, 21.9243) centre (0, 0) ccw
  arc A1027 (14.3045, 29.1827) -> (14.0967, 29.2836) centre (0, 0) ccw
  arc A1028 (15.6768, 28.469) -> (15.4741, 28.5797) centre (0, 0) ccw
  arc A1029 (17.0137, 27.6909) -> (16.8165, 27.8111) centre (0, 0) ccw
  arc A1030 (18.312, 26.85) -> (18.1207, 26.9794) centre (0, 0) ccw
  arc A1031 (19.5688, 25.9482) -> (19.384, 26.0866) centre (0, 0) ccw
  arc A1032 (20.7813, 24.9877) -> (20.6033, 25.1348) centre (0, 0) ccw
  arc A1033 (14.0889, 30.5365) -> (13.8517, 30.6449) centre (0, 0) ccw
  arc A1034 (15.5259, 29.8316) -> (15.2941, 29.9511) centre (0, 0) ccw
  arc A1035 (16.9278, 29.059) -> (16.702, 29.1894) centre (0, 0) ccw
  arc A1036 (18.2913, 28.2207) -> (18.0719, 28.3616) centre (0, 0) ccw
  arc A1037 (19.6134, 27.3184) -> (19.401, 27.4696) centre (0, 0) ccw
  arc A1038 (20.891, 26.3542) -> (20.686, 26.5154) centre (0, 0) ccw
  arc A1039 (22.1213, 25.3303) -> (21.9243, 25.5011) centre (0, 0) ccw
  arc A1040 (23.3015, 24.249) -> (23.1128, 24.429) centre (0, 0) ccw
  arc A1041 (24.429, 23.1128) -> (24.249, 23.3015) centre (0, 0) ccw
  arc A1042 (25.5011, 21.9243) -> (25.3303, 22.1213) centre (0, 0) ccw
  arc A1043 (26.5154, 20.686) -> (26.3542, 20.891) centre (0, 0) ccw
  arc A1044 (27.4696, 19.401) -> (27.3184, 19.6134) centre (0, 0) ccw
  arc A1045 (28.3616, 18.0719) -> (28.2207, 18.2913) centre (0, 0) ccw
  arc A1046 (29.9511, 15.2941) -> (29.8316, 15.5259) centre (0, 0) ccw
  arc A1047 (29.1894, 16.702) -> (29.059, 16.9278) centre (0, 0) ccw
  arc A1048 (29.2836, 14.0967) -> (29.1827, 14.3045) centre (0, 0) ccw
  arc A1049 (28.5797, 15.4741) -> (28.469, 15.6768) centre (0, 0) ccw
  arc A1050 (27.8111, 16.8165) -> (27.6909, 17.0137) centre (0, 0) ccw
  arc A1051 (26.9794, 18.1207) -> (26.85, 18.312) centre (0, 0) ccw
  arc A1052 (26.0866, 19.384) -> (25.9482, 19.5688) centre (0, 0) ccw
  arc A1053 (25.1348, 20.6033) -> (24.9877, 20.7813) centre (0, 0) ccw
  arc A1054 (24.1259, 21.7759) -> (23.9706, 21.9468) centre (0, 0) ccw
  arc A1055 (23.0625, 22.8992) -> (22.8992, 23.0625) centre (0, 0) ccw
  arc A1056 (21.9468, 23.9706) -> (21.7759, 24.1259) centre (0, 0) ccw
  dimension "d0" = 70
  dimension "d3" = 0.2
  dimension "d4" = 0.13
  dimension "d5" = 0.66
  dimension "d6" = 7.34
  dimension "d9" = 360
  constraints: 1584 point on circle, 793 centre point, 793 equal radius, 7 symmetric about line, 2 end point, 2 horizontal alignment, 2 tangent, 2 vertical alignment, 1 horizontal, 2641 other
  measures "d0" diameter of A0
  measures "d3" diameter of A2
  measures "d4" distance from line of L0 A2.centre
  measures "d5" distance from line of L0 A3.centre
  measures "d6" radius of A1
extrude "Extrusion1" add sketch "Sketch1" along normal blind 7
body "Solid1"
